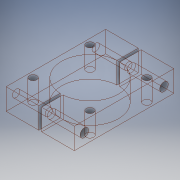
# Autodesk Inventor part: 4K heatsink bushing
Saved by Autodesk Inventor 2018 (Build 220112000, 112)
## iProperties
Created: 2019-03-19
Part Number: 4K heatsink bushing
Material: Copper
Document SubType Name: Modeling
Designer: freyja
Density: 8.94 g/cm^3
Appearance: Copper - Satin
Author: freyja
Autodesk Inventor part; units mm, degrees
note: some values were not read from the file. Chosen so that the rebuilt part matches the saved one: direction of "Hole3"; direction of "Hole4".
ref_plane "YZ Plane" through (0, 0, 0) normal (1, 0, 0) x (0, 1, 0)
ref_plane "XZ Plane" through (0, 0, 0) normal (0, 1, 0) x (-1, 0, 0)
ref_plane "XY Plane" through (0, 0, 0) normal (0, 0, 1) x (1, 0, 0)
sketch "Sketch8" plane through (0, 0, 0) normal (0, 1, 0) x (-1, 0, 0)
  circle A0 centre (0, 0) radius 12.7
  line L0 (-15.24, 22.225) -> (15.24, 22.225)
  line L1 (15.24, 22.225) -> (15.24, -22.225)
  line L2 (15.24, -22.225) -> (-15.24, -22.225)
  line L3 (-15.24, -22.225) -> (-15.24, 22.225)
  line L4 (-15.24, 22.225) -> (15.24, -22.225) construction
  line L5 (15.24, 22.225) -> (-15.24, -22.225) construction
  line L6 (-0.635, 22.225) -> (0.635, 22.225)
  line L7 (0.635, 22.225) -> (0.635, -22.225)
  line L8 (0.635, -22.225) -> (-0.635, -22.225)
  line L9 (-0.635, -22.225) -> (-0.635, 22.225)
  line L10 (-0.635, 22.225) -> (0.635, -22.225) construction
  line L11 (0.635, 22.225) -> (-0.635, -22.225) construction
  dimension "d34" = 25.4
  dimension "d35" = 30.48
  dimension "d36" = 44.45
  dimension "d37" = 1.27
  constraints: 24 end point, 4 midpoint, 4 parallel, 2 horizontal, 2 perpendicular, 1 centre point, 1 coincident, 1 point on line
  measures "d34" diameter of A0
  measures "d35" distance of L1.end L2.end
  measures "d36" distance of L0.end L1.end
  measures "d37" distance of L7.end L8.end
extrude "Extrusion6" add sketch "Sketch8" along normal blind 9.525 contours A0 L7 L0 L1 L2 | A0 L9 L2 L3 L0
sketch "Sketch9" plane through (15.24, 0, 22.225) normal (1, 0, 0) x (0, 0, -1)
  line L0 (4.445, -4.7625) -> (40.005, -4.7625) construction
  line L1 (40.005, -4.7625) -> (40.005, 4.7625) construction
  line L2 (40.005, 4.7625) -> (4.445, 4.7625) construction
  line L3 (4.445, 4.7625) -> (4.445, -4.7625) construction
  line L4 (4.445, -4.7625) -> (40.005, 4.7625) construction
  line L5 (40.005, -4.7625) -> (4.445, 4.7625) construction
  point P0 (22.225, 0)
  dimension "d40" = 35.56
  dimension "d41" = 9.525
  constraints: 12 end point, 2 coincident, 2 midpoint, 2 parallel, 1 horizontal, 1 perpendicular
  measures "d40" distance of L2.end L1.end
  measures "d41" distance of L1.end L0.end
hole "Hole3" at (15.24, 4.7625, 17.78) at (15.24, 4.7625, -17.78) direction (-1, 0, 0) diameter 3.81 depth 14.605 clearance for "Flat Head Machine Screw (82)" size "#6" standard "Ansi Unified Screw Threads"
sketch "Sketch10" plane through (-0.635, 0, 12.6841) normal (1, 0, 0) x (0, 0, -1)
  circle A0 centre (-5.0959, 4.7625) radius 1.905 projected
  circle A1 centre (30.4641, 4.7625) radius 1.905 projected
  point P0 (12.6841, 0)
  constraints: 2 coincident
hole "Hole4" at (-0.635, 4.7625, 17.78) at (-0.635, 4.7625, -17.78) direction (-1, 0, 0) diameter 3.302 end up to surface thread size "8-32 UNC" class "2B" standard "ANSI Unified Screw Threads"
sketch "Sketch11" plane through (0, 9.525, 0) normal (0, 1, 0) x (1, 0, 0)
  line L0 (-12.7, -12.7) -> (12.7, -12.7) construction
  line L1 (12.7, -12.7) -> (12.7, 12.7) construction
  line L2 (12.7, 12.7) -> (-12.7, 12.7) construction
  line L3 (-12.7, 12.7) -> (-12.7, -12.7) construction
  line L4 (-12.7, -12.7) -> (12.7, 12.7) construction
  line L5 (12.7, -12.7) -> (-12.7, 12.7) construction
  point P0 (0, 0)
  dimension "d56" = 25.4
  dimension "d57" = 25.4
  constraints: 12 end point, 4 coincident, 2 midpoint, 2 parallel, 1 horizontal, 1 perpendicular
  measures "d56" distance of L2.end L1.end
  measures "d57" distance of L1.end L0.end
hole "Hole5" at (-12.7, 9.525, -12.7) at (12.7, 9.525, -12.7) at (12.7, 9.525, 12.7) at (-12.7, 9.525, 12.7) direction (0, -1, 0) diameter 3.302 end through all thread size "8-32 UNC" class "2B" standard "ANSI Unified Screw Threads"
body "Solid2"
